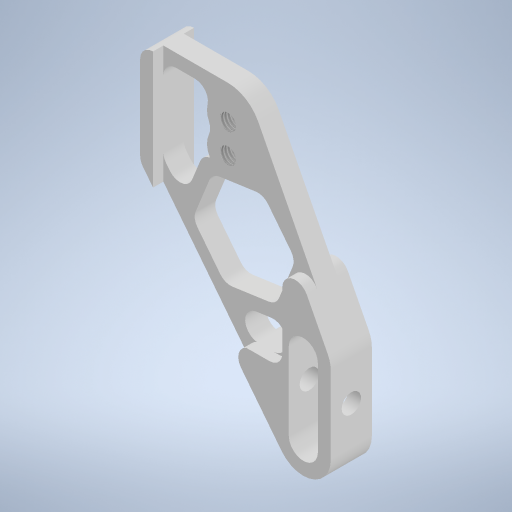
# Autodesk Inventor part: VerticalSlideMiddleBottomHexagonPocket2.2
Saved by Autodesk Inventor 2023 (Build 270158000, 158)
## iProperties
Created: 2022-10-14
Part Number: VerticalSlideMiddleBottomHexagonPocket2.2
Material: Generic
Document SubType Name: Modeling
Designer: deli
Density: 1 g/cm^3
Appearance: Default
Mass: 2.89315 g
Surface Area: 26.1343 cm^2
Volume: 2.89315 cm^3
Author: deli
Autodesk Inventor part; units mm, degrees
ref_plane "YZ Plane" through (0, 0, 0) normal (1, 0, 0) x (0, 1, 0)
ref_plane "XZ Plane" through (0, 0, 0) normal (0, 1, 0) x (-1, 0, 0)
ref_plane "XY Plane" through (0, 0, 0) normal (0, 0, 1) x (1, 0, 0)
sketch "Sketch1" plane through (0, 0, 0) normal (0, 0, 1) x (1, 0, 0)
  line L0 (-75.1619, -151.2747) -> (-75.1619, -164.2747)
  line L1 (-74.7357, -165.5089) -> (-53.2562, -192.8974)
  circle A0 centre (-63.1619, -159.0247) radius 1.25
  circle A1 centre (-63.1619, -154.5247) radius 1.25
  arc A2 (-52.1619, -190.2747) -> (-47.6619, -190.2747) centre (-49.9119, -190.2747) ccw
  arc A3 (-47.6619, -178.2747) -> (-52.1619, -178.2747) centre (-49.9119, -178.2747) ccw
  line L2 (-47.6619, -178.2747) -> (-47.6619, -190.2747)
  line L3 (-52.1619, -178.2747) -> (-52.1619, -190.2747)
  line L4 (-45.6619, -178.2747) -> (-45.6619, -190.2747)
  arc A4 (-53.2562, -192.8974) -> (-45.6619, -190.2747) centre (-49.9119, -190.2747) ccw
  arc A5 (-45.6619, -178.2747) -> (-46.1268, -176.3419) centre (-49.9119, -178.2747) ccw
  line L5 (-46.1268, -176.3419) -> (-58.4862, -152.1372)
  line L6 (-73.1619, -149.2747) -> (-63.1619, -149.2747)
  arc A6 (-58.4862, -152.1372) -> (-63.1619, -149.2747) centre (-63.1619, -154.5247) ccw
  arc A7 (-73.1619, -149.2747) -> (-75.1619, -151.2747) centre (-73.1619, -151.2747) ccw
  arc A8 (-75.1619, -164.2747) -> (-74.7357, -165.5089) centre (-73.1619, -164.2747) ccw
  line L7 (-52.1619, -182.7747) -> (-56.1619, -182.7747)
  line L8 (-56.1619, -182.7747) -> (-56.1619, -185.7747)
  line L9 (-56.1619, -185.7747) -> (-52.1619, -185.7747)
  point P0 (0, 0)
  dimension "d2" = 2.5
  dimension "d11" = 2
  dimension "d22" = 12
  dimension "d46" = 2
  dimension "d47" = 4.5
  dimension "d84" = 4
  dimension "d86" = 12
  dimension "d87" = 12
  dimension "d88" = 23
  dimension "d90" = 4
  dimension "d91" = 3
  dimension "d92" = 4.5
  dimension "d94" = 15
  dimension "d95" = 19.25
  dimension "d96" = 2
  constraints: 20 end point, 16 point on circle, 13 tangent, 9 centre point, 4 equal radius, 4 point on line, 3 perpendicular, 2 coincident, 2 vertical, 1 concentric, 1 horizontal, 1 parallel
  measures "d2" diameter of A0
  measures "d22" distance of A2.centre A3.centre
  measures "d46" radial gap between concentric circles of A4 A2
  measures "d47" distance between parallel lines of L2 L3
  measures "d84" distance edge to line of A1 L6
  measures "d86" distance from line of A1.centre L0
  measures "d87" distance from line of A0.centre L0
  measures "d88" distance between parallel lines of L3 L0
  measures "d90" distance of L7.start L7.end
  measures "d91" distance of L7.end L8.end
  measures "d92" distance from line of L3.start L7
  measures "d94" distance from line of L6 L0.end
  measures "d95" vertical distance of A3.centre A0.centre
  measures "d96" radius of A7
extrude "Extrusion1" add sketch "Sketch1" along normal blind 6.35 contours A7 L6 A6 L5 A5 L4 A4 L1 A8 L0 | L9 L8 L7 L3
thread "Thread2" size "M3x0.5" class "6H" standard "ANSI Metric M Profile" full length
thread "Thread6" size "M3x0.5" class "6H" standard "ANSI Metric M Profile" full length
sketch "Sketch8" plane through (-52.1619, -190.2747, 0) normal (1, 0, 0) x (0, 0, -1)
  line L0 (0, 0) -> (0, 12) construction
  line L1 (0, 12) -> (-6.35, 12) construction
  line L2 (-6.35, 0) -> (-6.35, 12) construction
  line L3 (0, 0) -> (-6.35, 0) construction
  line L4 (0, 0) -> (-6.35, 0) construction
  line L5 (-6.35, 12) -> (0, 0) construction
  line L6 (-6.35, 0) -> (0, 12) construction
  circle A0 centre (-3.175, 6) radius 1.5
  point P0 (0, 190.2747)
  dimension "d97" = 3
  constraints: 4 end point, 1 centre point, 1 midpoint
  measures "d97" diameter of A0
extrude "Extrusion7" cut sketch "Sketch8" along normal blind 10 and the other way blind 4
sketch "Sketch12" plane through (0, 0, 6.35) normal (0, 0, 1) x (1, 0, 0)
  line L0 (-75.1619, -151.2747) -> (-75.1619, -164.2747) projected
  arc A0 (-75.1619, -164.2747) -> (-74.7357, -165.5089) centre (-73.1619, -164.2747) ccw projected
  line L1 (-74.7357, -165.5089) -> (-53.2562, -192.8974) projected
  arc A1 (-53.2562, -192.8974) -> (-45.6619, -190.2747) centre (-49.9119, -190.2747) ccw projected
  line L2 (-45.6619, -190.2747) -> (-45.6619, -178.2747) projected
  arc A2 (-45.6619, -178.2747) -> (-46.1268, -176.3419) centre (-49.9119, -178.2747) ccw projected
  line L3 (-46.1268, -176.3419) -> (-58.4862, -152.1372) projected
  arc A3 (-58.4862, -152.1372) -> (-63.1619, -149.2747) centre (-63.1619, -154.5247) ccw projected
  line L4 (-63.1619, -149.2747) -> (-73.1619, -149.2747) projected
  arc A4 (-73.1619, -149.2747) -> (-75.1619, -151.2747) centre (-73.1619, -151.2747) ccw projected
  circle A5 centre (-63.1619, -159.0247) radius 1.25 projected
  circle A6 centre (-63.1619, -154.5247) radius 1.25 projected
  line L5 (-47.6619, -178.2747) -> (-47.6619, -190.2747) projected
  arc A7 (-52.1619, -190.2747) -> (-47.6619, -190.2747) centre (-49.9119, -190.2747) ccw projected
  line L6 (-52.1619, -190.2747) -> (-52.1619, -178.2747) projected
  arc A8 (-47.6619, -178.2747) -> (-52.1619, -178.2747) centre (-49.9119, -178.2747) ccw projected
  line L7 (-73.1619, -164.2747) -> (-73.1619, -151.2747)
  line L8 (-73.1619, -151.2747) -> (-63.1619, -151.2747)
  line L9 (-54.1619, -176.7964) -> (-54.1619, -181.7747)
  arc A9 (-63.1619, -151.2747) -> (-65.5072, -156.7747) centre (-63.1619, -154.5247) ccw
  arc A10 (-60.8167, -156.7747) -> (-60.2675, -153.0467) centre (-63.1619, -154.5247) ccw
  arc A11 (-45.6619, -178.2747) -> (-46.1268, -176.3419) centre (-49.9119, -178.2747) ccw
  arc A12 (-49.5477, -174.0403) -> (-54.1619, -178.2747) centre (-49.9119, -178.2747) ccw
  line L10 (-68.5958, -170.0969) -> (-65.6052, -162.6554)
  line L11 (-65.6052, -162.6554) -> (-57.6653, -161.5246)
  line L12 (-57.6653, -161.5246) -> (-52.7161, -167.8354)
  line L13 (-52.7161, -167.8354) -> (-55.7067, -175.2769)
  line L14 (-55.7067, -175.2769) -> (-63.6466, -176.4077)
  line L15 (-63.6466, -176.4077) -> (-68.5958, -170.0969)
  line L16 (-67.0303, -160.8382) -> (-70.021, -168.2797)
  line L17 (-62.2214, -178.2249) -> (-54.1619, -177.0771)
  line L18 (-70.021, -168.2797) -> (-73.1619, -164.2747)
  line L19 (-58.1619, -183.4011) -> (-62.2214, -178.2249)
  line L20 (-63.6466, -176.4077) -> (-68.5958, -170.0969)
  line L21 (-57.0171, -159.4121) -> (-60.0157, -159.8392)
  line L22 (-65.9557, -160.6852) -> (-67.0303, -160.8382)
  arc A13 (-65.5072, -156.7747) -> (-65.9557, -160.6852) centre (-63.1619, -159.0247) ccw
  arc A14 (-60.0157, -159.8392) -> (-60.8167, -156.7747) centre (-63.1619, -159.0247) ccw
  line L23 (-60.2675, -153.0467) -> (-57.0171, -159.4121)
  line L24 (-51.5099, -170.1975) -> (-49.5477, -174.0403)
  line L25 (-54.1619, -176.7964) -> (-51.5099, -170.1975)
  line L26 (-53.4693, -175.0728) -> (-53.0875, -175.4501)
  line L27 (-52.1619, -181.7747) -> (-58.1619, -181.7747)
  line L28 (-58.1619, -181.7747) -> (-58.1619, -186.7747)
  line L29 (-58.1619, -186.7747) -> (-52.1619, -186.7747)
  line L30 (-52.1619, -186.7747) -> (-52.1619, -181.7747)
  point P0 (0, 0)
  point P1 (-54.1619, -188.5015)
  point P2 (-60.656, -168.9661)
  dimension "d109" = 2
  dimension "d112" = 2
  dimension "d113" = 2
  dimension "d115" = 2
  dimension "d117" = 2
  dimension "d118" = 2
  dimension "d119" = 2
  dimension "d120" = 3.25
  dimension "d121" = 2
  dimension "d122" = 2
  dimension "d123" = 2
  dimension "d124" = 2
  dimension "d125" = 2
  dimension "d126" = 2
  dimension "d130" = 6
  dimension "d131" = 5
  dimension "d132" = 3.5
  constraints: 49 end point, 13 point on circle, 8 point on line, 6 centre point, 3 collinear, 2 equal radius, 2 parallel, 1 horizontal, 1 perpendicular, 1 tangent, 14 other
  measures "d109" distance between parallel lines of L6 L9
  measures "d112" radial gap between concentric circles of A6 A9
  measures "d113" radial gap between concentric circles of A12 A8
  measures "d115" distance between parallel lines of L0 L7
  measures "d117" distance between parallel lines of L18 L1
  measures "d118" distance between parallel lines of L10 L16
  measures "d119" distance from line of L3 L12.end
  measures "d120" distance from line of A5.centre L11
  measures "d121" distance between parallel lines of L11 L22
  measures "d122" distance between parallel lines of L21 L11
  measures "d123" distance between parallel lines of L3 L23
  measures "d124" distance between parallel lines of L14 L17
  measures "d125" distance between parallel lines of L25 L13
  measures "d126" distance between parallel lines of L3 L24
  measures "d130" distance of L29.end L28.end
  measures "d131" distance of L27.end L28.end
  measures "d132" distance from line of L27 A2.centre
extrude "Extrusion10" cut sketch "Sketch12" against normal blind 10 contours L19 L17 L9 L27 L28 | L7 L8 A9 A13 L22 L16 L18 | L10 L11 L12 L13 L14 L15
fillet "Fillet6" radius 2 17 edges at (-62.2214, -178.2249, 3.175) (-58.1619, -183.4011, 3.175) (-58.1619, -181.7747, 3.175) (-54.1619, -181.7747, 3.175) (-54.1619, -177.0771, 3.175) (-63.6466, -176.4077, 3.175) (-55.7067, -175.2769, 3.175) (-52.7161, -167.8354, 3.175) (-57.6653, -161.5246, 3.175) (-65.6052, -162.6554, 3.175) (-68.5958, -170.0969, 3.175) (-70.021, -168.2797, 3.175) (-67.0303, -160.8382, 3.175) (-73.1619, -164.2747, 3.175) (-73.1619, -151.2747, 3.175) (-63.1619, -151.2747, 3.175) (-65.5072, -156.7747, 3.175)
sketch "Sketch13" plane through (0, 0, 6.35) normal (0, 0, 1) x (1, 0, 0)
  line L0 (-73.1619, -145.0083) -> (-53.1619, -145.0083)
  line L1 (-53.1619, -145.0083) -> (-53.1619, -181.7747)
  line L2 (-53.1619, -181.7747) -> (-73.1619, -181.7747)
  line L3 (-73.1619, -181.7747) -> (-73.1619, -145.0083)
  line L4 (-75.1619, -151.2747) -> (-75.1619, -164.2747) projected
  line L5 (-56.1619, -181.7747) -> (-58.0429, -181.7747) projected
  line L6 (-52.1619, -190.2747) -> (-52.1619, -178.2747) projected
  circle A0 centre (-51.1619, -170.879) radius 2
  line L7 (-46.1268, -176.3419) -> (-58.4862, -152.1372) projected
  point P0 (0, 0)
  point P1 (-49.3807, -169.9695)
  point P2 (-53.1619, -162.5643)
  point P3 (-53.1619, -170.879)
  dimension "d134" = 2
  dimension "d135" = 1
  dimension "d140" = 4
  constraints: 8 end point, 2 parallel, 2 tangent, 1 centre point, 1 collinear, 1 horizontal, 1 perpendicular
  measures "d134" distance between parallel lines of L4 L3
  measures "d135" distance between parallel lines of L6 L1
  measures "d140" diameter of A0
extrude "Extrusion11" cut sketch "Sketch13" against normal blind 1.5875 contours L0 L1 L2 L3 | L7 A0 L1
sketch "Sketch14" plane through (0, 0, 0) normal (0, 0, -1) x (-1, 0, 0)
  circle A0 centre (63.1619, -159.0247) radius 1.25 projected
  circle A1 centre (63.1619, -154.5247) radius 1.25 projected
  arc A2 (53.4287, -166.9268) -> (53.1467, -168.9068) centre (55.0024, -168.161) ccw projected
  line L0 (53.1619, -170.879) -> (53.1619, -181.7747) projected
  line L1 (58.4862, -152.1372) -> (49.3807, -169.9695) projected
  arc A3 (63.1619, -149.2747) -> (58.4862, -152.1372) centre (63.1619, -154.5247) ccw projected
  line L2 (73.1619, -149.2747) -> (63.1619, -149.2747) projected
  line L3 (73.1619, -153.2747) -> (73.1619, -149.2747) projected
  arc A4 (73.1619, -153.2747) -> (71.1619, -151.2747) centre (71.1619, -153.2747) ccw projected
  line L4 (68.261, -151.2747) -> (71.1619, -151.2747) projected
  arc A5 (68.261, -151.2747) -> (66.3185, -153.7509) centre (68.261, -153.2747) ccw projected
  arc A6 (66.0983, -155.9175) -> (66.3185, -153.7509) centre (63.1619, -154.5247) ccw projected
  arc A7 (66.0983, -155.9175) -> (66.0983, -157.6318) centre (67.9054, -156.7747) ccw projected
  arc A8 (65.9557, -160.6852) -> (66.0983, -157.6318) centre (63.1619, -159.0247) ccw projected
  arc A9 (67.4604, -161.9083) -> (65.9557, -160.6852) centre (65.6046, -162.6541) ccw projected
  line L5 (68.7292, -165.0655) -> (67.4604, -161.9083) projected
  arc A10 (68.7292, -165.0655) -> (72.1587, -165.5539) centre (70.585, -164.3197) ccw projected
  line L6 (72.7357, -164.8182) -> (72.1587, -165.5539) projected
  arc A11 (72.7357, -164.8182) -> (73.1619, -163.5839) centre (71.1619, -163.5839) ccw projected
  line L7 (73.1619, -167.5156) -> (73.1619, -163.5839) projected
  line L8 (61.9792, -181.7747) -> (73.1619, -167.5156) projected
  line L9 (58.7344, -181.7747) -> (61.9792, -181.7747) projected
  arc A12 (58.7344, -181.7747) -> (60.0219, -181.0295) centre (58.4482, -179.7953) ccw projected
  line L10 (60.0837, -180.9507) -> (60.0219, -181.0295) projected
  arc A13 (60.0837, -180.9507) -> (58.7919, -177.7365) centre (58.51, -179.7165) ccw projected
  line L11 (56.4439, -177.4021) -> (58.7919, -177.7365) projected
  arc A14 (56.4439, -177.4021) -> (54.1619, -179.3821) centre (56.1619, -179.3821) ccw projected
  line L12 (54.1619, -179.7747) -> (54.1619, -179.3821) projected
  arc A15 (54.1619, -179.7747) -> (56.1619, -181.7747) centre (56.1619, -179.7747) ccw projected
  line L13 (53.1619, -181.7747) -> (56.1619, -181.7747) projected
  line L14 (55.2761, -174.2055) -> (53.1467, -168.9068) projected
  arc A16 (55.2761, -174.2055) -> (56.8499, -175.4397) centre (57.1319, -173.4597) ccw projected
  line L15 (62.5034, -176.2449) -> (56.8499, -175.4397) projected
  arc A17 (62.5034, -176.2449) -> (64.3592, -175.4991) centre (62.7854, -174.2648) ccw projected
  line L16 (67.8832, -171.0055) -> (64.3592, -175.4991) projected
  arc A18 (67.8832, -171.0055) -> (68.1652, -169.0255) centre (66.3095, -169.7713) ccw projected
  line L17 (66.0358, -163.7268) -> (68.1652, -169.0255) projected
  arc A19 (66.0358, -163.7268) -> (64.462, -162.4926) centre (64.18, -164.4726) ccw projected
  line L18 (58.8085, -161.6874) -> (64.462, -162.4926) projected
  arc A20 (58.8085, -161.6874) -> (56.9527, -162.4332) centre (58.5265, -163.6675) ccw projected
  line L19 (53.4287, -166.9268) -> (56.9527, -162.4332) projected
  arc A21 (53.1619, -170.879) -> (49.3807, -169.9695) centre (51.1619, -170.879) ccw projected
  point P0 (0, 0)
extrude "Extrusion12" cut sketch "Sketch14" against normal blind 1.5875
fillet "Fillet7" radius 2 4 edges at (-61.9792, -181.7747, 5.5562) (-53.1619, -181.7747, 5.5562) (-53.1619, -181.7747, 0.7937) (-61.9792, -181.7747, 0.7937)
equation "\"d22\" = d17"
equation "\"d17\" = 12"
body "Solid1"
